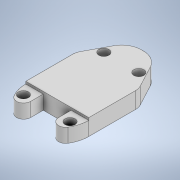
# Autodesk Inventor part: finger_mount
Saved by Autodesk Inventor 2021.1 (Build 251245010, 245A)
## iProperties
Created: 2021-06-02
Part Number: finger_mount
Material: Generic
Document SubType Name: Modeling
Designer: fraaw
Density: 1 g/cm^3
Appearance: Default
Author: fraaw
Autodesk Inventor part; units mm, degrees
ref_plane "YZ Plane" through (0, 0, 0) normal (1, 0, 0) x (0, 1, 0)
ref_plane "XZ Plane" through (0, 0, 0) normal (0, 1, 0) x (-1, 0, 0)
ref_plane "XY Plane" through (0, 0, 0) normal (0, 0, 1) x (1, 0, 0)
sketch "Sketch1" plane through (0, 0, 0) normal (0, 1, 0) x (-1, 0, 0)
  line L0 (13.5, 17.5) -> (-13.5, 17.5)
  line L1 (-13.5, 17.5) -> (-13.5, -17.5)
  line L2 (-13.5, -17.5) -> (13.5, -17.5) construction
  line L3 (13.5, -17.5) -> (13.5, 17.5)
  line L4 (13.5, 17.5) -> (-13.5, -17.5) construction
  line L5 (-13.5, 17.5) -> (13.5, -17.5) construction
  line L6 (0, 17.5) -> (0, -33.821) construction
  line L7 (13.5, -17.5) -> (5.5, -32.5)
  line L8 (5.5, -32.5) -> (0, -32.5)
  line L9 (-13.5, -17.5) -> (-5.5, -32.5)
  line L10 (-5.5, -32.5) -> (0, -32.5)
  point P0 (0, 0)
  dimension "d0" = 5.5
  dimension "d1" = 35
  dimension "d2" = 27
  dimension "d3" = 15
  constraints: 22 end point, 3 midpoint, 2 parallel, 2 perpendicular, 1 horizontal, 1 point on line, 1 symmetric about line, 1 vertical
  measures "d0" distance of L7.end L8.end
  measures "d1" distance of L2.end L0.start
  measures "d2" distance of L0.start L0.end
  measures "d3" distance between parallel lines of L2 L8
extrude "Extrusion1" add sketch "Sketch1" along normal blind 7
fillet "Fillet1" radius 8.5 2 edges at (5.5, 3.5, -32.5) (-5.5, 3.5, -32.5)
fillet "Fillet2" radius 5.5 2 edges at (13.5, 3.5, -17.5) (-13.5, 3.5, -17.5)
fillet "Fillet3" radius 13.5 2 edges at (-13.5, 3.5, 17.5) (13.5, 3.5, 17.5)
sketch "Sketch2" plane through (0, 7, 0) normal (0, 1, 0) x (1, 0, 0)
  line L0 (-13.5, 16.125) -> (-13.5, -4) projected
  arc A0 (-13.5, -4) -> (13.5, -4) centre (0, -4) ccw projected
  line L1 (-13.5, -4) -> (13.5, -4)
  line L2 (13.5, -4) -> (13.5, -17.5)
  line L3 (13.5, -17.5) -> (-13.5, -17.5)
  line L4 (-13.5, -17.5) -> (-13.5, -4)
  point P0 (0, 0)
  constraints: 8 end point, 2 parallel, 1 horizontal, 1 perpendicular
extrude "Extrusion2" cut sketch "Sketch2" against normal blind 1
sketch "Sketch3" plane through (0, 6, 0) normal (0, 1, 0) x (1, 0, 0)
  line L0 (-13.5, -4) -> (13.5, -4) projected
  line L1 (0, -4) -> (0, -30.3516) construction
  line L2 (-6, -17.5) -> (6, -17.5)
  line L3 (6, -17.5) -> (6, -4)
  line L4 (6, -4) -> (-6, -4)
  line L5 (-6, -4) -> (-6, -17.5)
  line L6 (-6, -17.5) -> (6, -4) construction
  line L7 (6, -17.5) -> (-6, -4) construction
  arc A0 (-13.5, -4) -> (13.5, -4) centre (0, -4) ccw projected
  point P0 (0, 0)
  point P1 (0, -10.75)
  point P2 (-6, -16.0934)
  point P3 (6, -16.0934)
  dimension "d11" = 12
  constraints: 14 end point, 3 midpoint, 2 parallel, 2 point on line, 1 horizontal, 1 perpendicular, 1 tangent, 1 vertical
  measures "d11" distance of L2.start L2.end
extrude "Extrusion3" cut sketch "Sketch3" against normal up to next contours L0 L3 A0 L5
sketch "Sketch4" plane through (0, 0, 0) normal (0, -1, 0) x (1, 0, 0)
  line L0 (0, -29.5282) -> (0, 0) construction
  line L1 (-13.5, 4) -> (13.5, 4) projected
  line L2 (0.4, -32.5) -> (-0.4, -32.5) projected
  point P0 (7.5, -23.5)
  point P1 (10, 8.5)
  point P2 (-7.5, -23.5)
  point P3 (-10, 8.5)
  dimension "d14" = 32
  dimension "d15" = 9
  dimension "d16" = 7.5
  dimension "d17" = 10
  constraints: 2 end point, 2 symmetric about line, 1 perpendicular
  measures "d14" vertical distance of point (10, 8.5) point (7.5, -23.5)
  measures "d15" distance from line of point (7.5, -23.5) L2
  measures "d16" distance from line of L0 point (7.5, -23.5)
  measures "d17" distance from line of L0 point (10, 8.5)
hole "Hole1" at (7.5, 0, -23.5) at (10, 0, 8.5) at (-10, 0, 8.5) at (-7.5, 0, -23.5) direction (0, 1, 0) diameter 2.3 depth 7 tip angle 118
sketch "Sketch5" plane through (0, 7, 0) normal (0, 1, 0) x (1, 0, 0)
  circle A0 centre (-7.5, 23.5) radius 1.15 projected
  circle A1 centre (-7.5, 23.5) radius 2.15
  circle A2 centre (7.5, 23.5) radius 1.15 projected
  circle A3 centre (7.5, 23.5) radius 2.15
  point P0 (0, 0)
  dimension "d25" = 4.3
  dimension "d26" = 4.3
  constraints: 2 centre point, 2 coincident
  measures "d25" diameter of A1
  measures "d26" diameter of A3
extrude "Extrusion4" cut sketch "Sketch5" against normal blind 3 contours A0 | A1 | A2 | A3
sketch "Sketch6" plane through (0, 6, 0) normal (0, 1, 0) x (1, 0, 0)
  circle A0 centre (-10, -8.5) radius 1.15 projected
  circle A1 centre (-10, -8.5) radius 2.15
  circle A2 centre (10, -8.5) radius 1.15 projected
  circle A3 centre (10, -8.5) radius 2.15
  point P0 (0, 0)
  dimension "d29" = 4.3
  dimension "d30" = 4.3
  constraints: 2 centre point, 2 coincident
  measures "d29" diameter of A1
  measures "d30" diameter of A3
extrude "Extrusion5" cut sketch "Sketch6" against normal blind 3 contours A0 | A1 | A2 | A3
fillet "Fillet4" radius 3 2 edges at (-6, 3, 16.0934) (6, 3, 16.0934)
body "Solid1"
